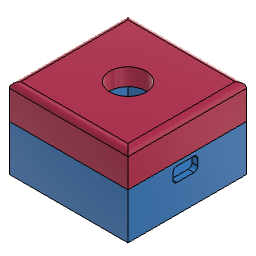
enclosureModel (Autodesk Fusion 360 design; units mm, degrees)
Autodesk Fusion 360 part; units mm, degrees
note: some values were not read from the file. Set by a fixed rule: which sketch regions a step uses.
sketch "base" plane through (0, 0, 0) normal (0, 0, 1) x (1, 0, 0)
  line L0 (0, 0) -> (62, 0)
  line L1 (62, 0) -> (62, 62)
  line L2 (62, 62) -> (0, 62)
  line L3 (0, 62) -> (0, 0)
  dimension "d1" = 62
  dimension "d2" = 62
  constraint horizontal L0
  constraint vertical L1
  constraint horizontal L2
  constraint vertical L3
  constraint coincident L0.start L3.end
  measures "d1" distance of L0.start L0.end
  measures "d2" distance of L0.start L2.end
extrude "Extrude1" add sketch "base" along normal blind 24 makes body 1
sketch "walls" plane through (0, 0, 24) normal (0, 0, 1) x (-1, 0, 0)
  line L0 (0, -62) -> (0, 0)
  line L1 (0, 0) -> (-62, 0)
  line L2 (-62, 0) -> (-62, -62)
  line L3 (-62, -62) -> (0, -62)
  line L4 (-3, -59) -> (-59, -59)
  line L5 (-59, -59) -> (-59, -3)
  line L6 (-59, -3) -> (-3, -3)
  line L7 (-3, -3) -> (-3, -59)
  dimension "d5" = 56
  dimension "d6" = 56
  dimension "d7" = 3
  dimension "d8" = 3
  constraint horizontal L4
  constraint vertical L5
  constraint horizontal L6
  constraint vertical L7
  measures "d5" distance of L4.start L4.end
  measures "d6" distance of L4.start L6.end
  measures "d7" distance of L0 L4.start
  measures "d8" distance of L0.start L4
extrude "Extrude2" cut sketch "walls" against normal blind 19 contours L4 L5 L6 L7 bodies 1
sketch "base (1)" plane through (0, 0, 0) normal (0, 0, 1) x (1, 0, 0)
  line L0 (0, 0) -> (62, 0)
  line L1 (62, 0) -> (62, 62)
  line L2 (62, 62) -> (0, 62)
  line L3 (0, 62) -> (0, 0)
  dimension "d13" = 62
  dimension "d14" = 62
  constraint horizontal L0
  constraint vertical L1
  constraint horizontal L2
  constraint vertical L3
  constraint coincident L0.start L3.end
  measures "d13" distance of L0.start L0.end
  measures "d14" distance of L0.start L2.end
extrude "Extrude3" add sketch "base (1)" along normal blind 18 separate body makes body 2
sketch "walls (1)" plane through (0, 0, 0) normal (0, 0, -1) x (1, 0, 0)
  line L0 (0, 0) -> (0, -62)
  line L1 (0, -62) -> (62, -62)
  line L2 (62, -62) -> (62, 0)
  line L3 (62, 0) -> (0, 0)
  line L4 (3, -3) -> (59, -3)
  line L5 (59, -3) -> (59, -59)
  line L6 (59, -59) -> (3, -59)
  line L7 (3, -59) -> (3, -3)
  dimension "d17" = 56
  dimension "d18" = 56
  dimension "d19" = 3
  dimension "d20" = 3
  constraint horizontal L4
  constraint vertical L5
  constraint horizontal L6
  constraint vertical L7
  measures "d17" distance of L4.start L4.end
  measures "d18" distance of L4.start L6.end
  measures "d19" horizontal distance of L0.start L4.start
  measures "d20" vertical distance of L0.start L4.start
extrude "Extrude4" cut sketch "walls (1)" against normal blind 15 contours L4 L5 L6 L7 bodies 2
move_body "Move1" bodies 2 to x (1, 0, 0) y (0, 1, 0) z (0, 0, 1) at (0, 0, 24)
sketch "Sketch7" plane through (0, 0, 0) normal (1, 0, 0) x (0, 1, 0)
fillet "Fillet1" radius 3 1 faces at (20.6667, 41.3333, 42) on bodies 2
sketch "Sketch8" plane through (0, 0, 42) normal (0, 0, 1) x (-1, 0, 0)
  line L0 (-59, -3) -> (-59, -59)
  line L1 (-59, -59) -> (-3, -59)
  line L2 (-3, -59) -> (-3, -3)
  line L3 (-3, -3) -> (-59, -3)
hole "Hole1" at (31, 31, 42) direction (0, 0, -1) diameter 19 depth 8 tip angle 180 bodies 2
sketch "nixieHole" plane through (0, 0, 42) normal (0, 0, 1) x (1, 0, 0)
  circle A0 centre (31, 31) radius 9
  point P0 (0, 62)
  dimension "d28" = 18
  measures "d28" diameter of A0
extrude "Extrude5" add sketch "nixieHole" along normal blind 34 separate body makes body 3
sketch "Sketch10" plane through (0, 0, 76) normal (0, 0, 1) x (-1, 0, 0)
  circle A0 centre (-31, -31) radius 9
  circle A1 centre (-31, -31) radius 9
  dimension "d33" = 18
  constraint concentric A0 A1
  measures "d33" diameter of A1
extrude "Extrude6" add sketch "Sketch10" along normal blind 12 bodies 3
chamfer "Chamfer1" distance 7.5 angle 45 1 faces at (33.1816, 30.6117, 88) on bodies 3
extrude "Extrude7" add 1 faces at (31.3887, 30.5125, 88) along direction (0, 0, 1) blind 2 on bodies 3 bodies 3
chamfer "Chamfer2" distance 1 distance2 2 1 edges at (32.3985, 31.5424, 90) measured on face at (31.3887, 30.5125, 90) on bodies 3
sketch "usbHole" plane through (62, 0, 0) normal (1, 0, 0) x (0, 1, 0)
  line L0 (0, 0) -> (62, 0)
  line L1 (62, 0) -> (62, 24)
  line L2 (62, 24) -> (0, 24)
  line L3 (0, 24) -> (0, 0)
  line L4 (25.5, 22) -> (34.5, 22)
  line L5 (36.5, 20) -> (36.5, 16.6)
  line L6 (34.5, 14.6) -> (25.5, 14.6)
  line L7 (23.5, 16.6) -> (23.5, 20)
  arc A0 (25.5, 22) -> (23.5, 20) centre (25.5, 20) ccw
  arc A1 (23.5, 16.6) -> (25.5, 14.6) centre (25.5, 16.6) ccw
  arc A2 (34.5, 14.6) -> (36.5, 16.6) centre (34.5, 16.6) ccw
  arc A3 (36.5, 20) -> (34.5, 22) centre (34.5, 20) ccw
  point P0 (23.5, 22)
  point P1 (36.5, 22)
  point P2 (23.5, 14.6)
  dimension "d47" = 13
  dimension "d48" = 7.4
  dimension "d49" = 23.5
  dimension "d50" = 14.6
  dimension "d138" = 2
  constraint horizontal L4
  constraint vertical L5
  constraint horizontal L6
  constraint vertical L7
  constraint coincident P0 L4
  constraint coincident P0 L7
  constraint tangent L4 A0
  constraint tangent L7 A0
  constraint coincident P2 L7
  constraint coincident P2 L6
  constraint tangent L7 A1
  constraint tangent L6 A1
  constraint equal A0 A1
  constraint tangent L6 A2
  constraint tangent L5 A2
  constraint equal A0 A2
  constraint coincident P1 L5
  constraint coincident P1 L4
  constraint tangent L5 A3
  constraint tangent L4 A3
  constraint equal A0 A3
  measures "d47" distance of P0 P1
  measures "d48" distance of P0 P2
  measures "d49" distance of L3 L7
  measures "d50" distance of L0 L6
  measures "d138" radius of A0
extrude "Extrude9" cut sketch "usbHole" against normal blind 8 contours L4 L5 L6 L7 A0 A1 A2 A3 bodies 1
sketch "mountingHoles" plane through (0, 0, 5) normal (0, 0, 1) x (-1, 0, 0)
  line L0 (-59, -59) -> (-3, -59)
  line L1 (-3, -59) -> (-3, -3)
  line L2 (-3.5, -58.5) -> (-58.5, -58.5)
  line L3 (-58.5, -58.5) -> (-58.5, -3.5)
  line L4 (-58.5, -3.5) -> (-3.5, -3.5)
  line L5 (-3.5, -3.5) -> (-3.5, -58.5)
  line L6 (-8, -54) -> (-54, -54)
  line L7 (-54, -54) -> (-54, -8)
  line L8 (-54, -8) -> (-8, -8)
  line L9 (-8, -8) -> (-8, -54)
  line L10 (-3, -3) -> (-59, -3)
  line L11 (-59, -3) -> (-59, -59)
  dimension "d63" = 55
  dimension "d64" = 55
  dimension "d65" = 0.5
  dimension "d67" = 46
  dimension "d68" = 46
  dimension "d69" = 4.5
  dimension "d70" = 4.5
  dimension "d76" = 0.5
  constraint horizontal L2
  constraint vertical L3
  constraint horizontal L4
  constraint vertical L5
  constraint horizontal L6
  constraint vertical L7
  constraint horizontal L8
  constraint vertical L9
  measures "d63" distance of L2.start L2.end
  measures "d64" distance of L2.start L4.end
  measures "d65" distance of L1 L5
  measures "d67" distance of L6.start L6.end
  measures "d68" distance of L6.start L8.end
  measures "d69" distance of L4 L8
  measures "d70" distance of L3 L7
  measures "d76" distance of L4 L10
sketch "base (2)" plane through (0, 0, 0) normal (0, 0, 1) x (1, 0, 0)
  line L0 (58.5, 58.5) -> (3.5, 58.5)
  line L1 (3.5, 58.5) -> (3.5, 3.5)
  line L2 (3.5, 3.5) -> (58.5, 3.5)
  line L3 (58.5, 3.5) -> (58.5, 58.5)
  line L4 (0, 0) -> (62, 0)
  line L5 (62, 0) -> (62, 62)
  dimension "d87" = 55
  dimension "d88" = 55
  dimension "d89" = 3.5
  dimension "d90" = 3.5
  constraint horizontal L0
  constraint vertical L1
  constraint horizontal L2
  constraint vertical L3
  measures "d87" distance of L1.end L2.end
  measures "d88" distance of L0.start L2.end
  measures "d89" distance of L2 L4
  measures "d90" distance of L3 L5
extrude "Extrude12" add sketch "base (2)" along normal blind 1.6 separate body makes body 4
move_body "Move7" bodies 4 to x (1, 0, 0) y (0, 1, 0) z (0, 0, 1) at (0, 0, 15)
sketch "usbC" plane through (0, 0, 16.6) normal (0, 0, 1) x (-1, 0, 0)
  line L0 (-58.5, -3.5) -> (-58.5, -58.5)
  line L1 (-58.5, -58.5) -> (-3.5, -58.5)
  line L2 (-3.5, -58.5) -> (-3.5, -3.5)
  line L3 (-3.5, -3.5) -> (-58.5, -3.5)
  line L4 (-58.5, -26.5) -> (-50.5, -26.5)
  line L5 (-50.5, -26.5) -> (-50.5, -35.5)
  line L6 (-50.5, -35.5) -> (-58.5, -35.5)
  line L7 (-58.5, -35.5) -> (-58.5, -26.5)
  line L8 (-3.5, -3.5) -> (-58.5, -3.5)
  dimension "d93" = 23
  dimension "d94" = 8
  dimension "d95" = 9
  constraint horizontal L4
  constraint vertical L5
  constraint horizontal L6
  constraint vertical L7
  constraint coincident L0 L4.start
  measures "d93" distance of L4 L8
  measures "d94" distance of L4.start L4.end
  measures "d95" distance of L4.end L5.end
extrude "Extrude13" add sketch "usbC" along normal blind 4 contours L0 L4 L5 L6 L7 bodies 4
hole "Hole2" at (54, 8, 5) at (54, 54, 5) at (8, 54, 5) at (8, 8, 5) direction (0, 0, -1) diameter 6.5 depth 3 tip angle 180 bodies 1
extrude "Extrude14" add sketch "base (2)" along normal blind 1.6 separate body makes body 5
move_body "Move8" bodies 5 to x (1, 0, 0) y (0, 1, 0) z (0, 0, 1) at (0, 0, 28.6)
sketch "Sketch23" plane through (0, 0, 0) normal (0, 0, 1) x (1, 0, 0)
  line L0 (58.8, 3.2) -> (3.2, 3.2)
  line L1 (3.2, 3.2) -> (3.2, 58.8)
  line L2 (3.2, 58.8) -> (58.8, 58.8)
  line L3 (58.8, 58.8) -> (58.8, 3.2)
  line L4 (59, 3) -> (3, 3)
  line L5 (59, 59) -> (59, 3)
  dimension "d104" = 55.6
  dimension "d105" = 55.6
  dimension "d106" = 0.2
  dimension "d107" = 0.2
  constraint horizontal L0
  constraint vertical L1
  constraint horizontal L2
  constraint vertical L3
  measures "d104" distance of L0.start L0.end
  measures "d105" distance of L0.end L1.end
  measures "d106" distance of L0 L4
  measures "d107" distance of L3 L5
extrude "Extrude19" add sketch "Sketch23" along normal blind 32 separate body makes body 6
sketch "Sketch25" plane through (0, 0, 0) normal (0, 0, 1) x (1, 0, 0)
  line L0 (8.2, 8.2) -> (53.8, 8.2)
  line L1 (53.8, 8.2) -> (53.8, 53.8)
  line L2 (53.8, 53.8) -> (8.2, 53.8)
  line L3 (8.2, 53.8) -> (8.2, 8.2)
  line L4 (58.8, 3.2) -> (3.2, 3.2)
  line L5 (3.2, 3.2) -> (3.2, 58.8)
  line L6 (58.8, 58.8) -> (58.8, 3.2)
  line L7 (3.2, 58.8) -> (58.8, 58.8)
  dimension "d124" = 5
  dimension "d125" = 5
  dimension "d126" = 5
  dimension "d127" = 5
  constraint horizontal L0
  constraint vertical L1
  constraint horizontal L2
  constraint vertical L3
  measures "d124" distance of L0 L4
  measures "d125" distance of L3 L5
  measures "d126" distance of L1 L6
  measures "d127" distance of L2 L7
sketch "Sketch26" plane through (0, 0, 0) normal (0, 0, 1) x (1, 0, 0)
sketch "Sketch27" plane through (0, 0, 32) normal (0, 0, 1) x (-1, 0, 0)
  line L0 (-58.8, -58.8) -> (-3.2, -58.8)
  line L1 (-3.2, -58.8) -> (-3.2, -3.2)
  line L2 (-3.2, -3.2) -> (-58.8, -3.2)
  line L3 (-58.8, -3.2) -> (-58.8, -58.8)
  line L4 (-8.2, -53.8) -> (-53.8, -53.8)
  line L5 (-53.8, -53.8) -> (-53.8, -8.2)
  line L6 (-53.8, -8.2) -> (-8.2, -8.2)
  line L7 (-8.2, -8.2) -> (-8.2, -53.8)
  dimension "d132" = 5
  dimension "d133" = 5
  dimension "d134" = 5
  dimension "d135" = 5
  constraint horizontal L4
  constraint vertical L5
  constraint horizontal L6
  constraint vertical L7
  measures "d132" distance of L0 L4
  measures "d133" distance of L2 L6
  measures "d134" distance of L3 L5
  measures "d135" distance of L1 L7
extrude "Extrude22" cut sketch "Sketch27" against normal blind 32 contours L4 L5 L6 L7 bodies 6
move_body "Move10" bodies 6 to x (1, 0, 0) y (0, 1, 0) z (0, 0, 1) at (0, 0, 5)
sketch "Sketch28" plane through (0, 0, 39) normal (0, 0, -1) x (1, 0, 0)
  circle A0 centre (31, -31) radius 9.5
  line L0 (3, -59) -> (59, -59)
  line L1 (59, -59) -> (59, -3)
  line L2 (59, -3) -> (3, -3)
  line L3 (3, -3) -> (3, -59)
  circle A1 centre (31, -31) radius 11.5
  dimension "d139" = 23
  constraint concentric A0 A1
  measures "d139" diameter of A1
extrude "Extrude23" add sketch "Sketch28" along normal blind 6 contours A1 bodies 2
hidden bodies 3 4 5 6
named bodies: "Bottom", "Top", "Nixie", "PcbBottom", "PcbTop", "Helper"
